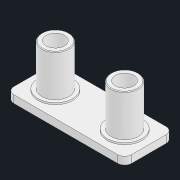
# Autodesk Inventor part: scara-base8
Saved by Autodesk Inventor 2022 (Build 260153000, 153)
## iProperties
Created: 2021-10-17
Part Number: scara-base8
Material: ABS プラスチック
Document SubType Name: Modeling
Designer: Yuta Kage
Density: 1.06 g/cm^3
Appearance: 滑らか - 白
Description: 印刷
Author: Yuta Kage
Autodesk Inventor part; units mm, degrees
ref_plane "YZ Plane" through (0, 0, 0) normal (1, 0, 0) x (0, 1, 0)
ref_plane "XZ Plane" through (0, 0, 0) normal (0, 1, 0) x (-1, 0, 0)
ref_plane "XY Plane" through (0, 0, 0) normal (0, 0, 1) x (1, 0, 0)
sketch "スケッチ1" plane through (0, 0, 0) normal (0, 1, 0) x (-1, 0, 0)
  line L0 (17, 7) -> (-17, 7)
  line L1 (-17, 7) -> (-17, -7)
  line L2 (-17, -7) -> (17, -7)
  line L3 (17, -7) -> (17, 7)
  line L4 (17, 7) -> (-17, -7) construction
  line L5 (-17, 7) -> (17, -7) construction
  point P0 (0, 0)
  dimension "d0" = 34
  dimension "d1" = 14
  constraints: 12 end point, 2 midpoint, 2 parallel, 1 horizontal, 1 perpendicular
  measures "d0" distance of L1.end L2.end
  measures "d1" distance of L2.end L0.start
extrude "押し出し1" add sketch "スケッチ1" along normal blind 2.2
sketch "スケッチ2" plane through (0, 2.2, 0) normal (0, 1, 0) x (1, 0, 0)
  circle A0 centre (-10, 0) radius 5
  circle A1 centre (10, 0) radius 5
  point P0 (0, 0)
  dimension "d4" = 10
  dimension "d5" = 10
  dimension "d6" = 10
  dimension "d7" = 10
  constraints: 2 centre point, 2 horizontal alignment
  measures "d4" diameter of A0
  measures "d5" diameter of A1
  measures "d6" distance of A0.centre point (0, 0)
  measures "d7" distance of point (0, 0) A1.centre
extrude "押し出し2" add sketch "スケッチ2" along normal blind 0.5
sketch "スケッチ3" plane through (-10, 2.7, 0) normal (0, 1, 0) x (1, 0, 0)
  circle A0 centre (0, 0) radius 5 projected
  circle A1 centre (20, 0) radius 5 projected
  circle A2 centre (0, 0) radius 3.95
  circle A3 centre (20, 0) radius 3.95
  point P0 (10, 0)
  dimension "d10" = 7.9
  dimension "d11" = 7.9
  constraints: 2 centre point, 2 coincident
  measures "d10" diameter of A2
  measures "d11" diameter of A3
extrude "押し出し3" add sketch "スケッチ3" along normal blind 12 contours A2 | A3
sketch "スケッチ5" plane through (-10, 14.7, 0) normal (0, 1, 0) x (1, 0, 0)
  circle A0 centre (0, 0) radius 3.95 projected
  circle A1 centre (20, 0) radius 3.95 projected
  point P0 (10, 0)
hole "穴2" at (10, 14.7, 0) at (-10, 14.7, 0) direction (0, -1, 0) diameter 5.3 end through all clearance for "Socket Head Cap Screw" size "M5" standard "Ansi Metric M Profile"
chamfer "面取り2" distance 0.2 angle 45 2 edges at (-13.95, 14.7, 0) (6.05, 14.7, 0)
fillet "フィレット2" radius 2 4 edges at (17, 1.1, 7) (17, 1.1, -7) (-17, 1.1, 7) (-17, 1.1, -7)
equation "\"d5\" = d4"
equation "\"d10\" = d11"
